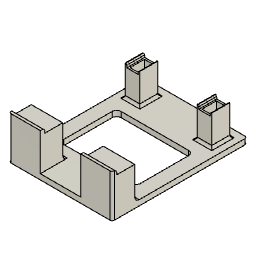
Header-Assembly-Jig (Autodesk Fusion 360 design; units mm, degrees)
Autodesk Fusion 360 part; units mm, degrees
sketch "Sketch1" plane through (0, 0, 0) normal (0, 0, 1) x (1, 0, 0)
  line L0 (1.9, -3.2) -> (-1.9, -3.2)
  line L1 (-1.9, -3.2) -> (-1.9, 3.2)
  line L2 (-1.9, 3.2) -> (1.9, 3.2)
  line L3 (1.9, 3.2) -> (1.9, -3.2)
  line L4 (1.9, -3.2) -> (-1.9, 3.2) construction
  line L5 (-1.9, -3.2) -> (1.9, 3.2) construction
  line L6 (2.55, -4) -> (-2.55, -4)
  line L7 (-2.55, -4) -> (-2.55, 4)
  line L8 (-2.55, 4) -> (2.55, 4)
  line L9 (2.55, 4) -> (2.55, -4)
  line L10 (2.55, -4) -> (-2.55, 4) construction
  line L11 (-2.55, -4) -> (2.55, 4) construction
  line L12 (3.25, -4) -> (-3.25, -4)
  line L13 (-3.25, -4) -> (-3.25, 4)
  line L14 (-3.25, 4) -> (3.25, 4)
  line L15 (3.25, 4) -> (3.25, -4)
  line L16 (3.25, -4) -> (-3.25, 4) construction
  line L17 (-3.25, -4) -> (3.25, 4) construction
  dimension "d1" = 3.8
  dimension "d2" = 6.4
  dimension "d3" = 5.1
  dimension "d4" = 8
  dimension "d5" = 6.5
  dimension "d6" = 8
  constraint horizontal L0
  constraint perpendicular L0 L1
  constraint parallel L0 L2
  constraint parallel L1 L3
  constraint coincident L4 origin
  constraint coincident L5 origin
  constraint horizontal L6
  constraint perpendicular L6 L7
  constraint parallel L6 L8
  constraint parallel L7 L9
  constraint coincident L10 origin
  constraint coincident L11 origin
  constraint horizontal L12
  constraint perpendicular L12 L13
  constraint parallel L12 L14
  constraint parallel L13 L15
  constraint coincident L16 origin
  constraint coincident L17 origin
  measures "d1" distance of L1.end L2.end
  measures "d2" distance of L0.end L1.end
  measures "d3" distance of L7.end L8.end
  measures "d4" distance of L6.end L7.end
  measures "d5" distance of L13.end L14.end
  measures "d6" distance of L12.end L13.end
extrude "Extrude1" add sketch "Sketch1" along normal blind 1.5 contours L9 L12 L14 L15 | L7 L12 L13 L14 makes body 1 at (3.25, 1.3333, 0.5) makes body 2 at (-3.25, -1.3333, 0.5)
extrude "Extrude2" add sketch "Sketch1" against normal blind 8 bodies 1 2
chamfer "Chamfer1" distance 0.5 angle 45 2 edges at (-2.55, 0, 1.5) (2.55, 0, 1.5) on bodies 1
sketch "Sketch2" plane through (0, 0, -8) normal (0, 0, -1) x (1, 0, 0)
  line L0 (1.9, -3.2) -> (-1.9, -3.2)
  line L1 (-1.9, -3.2) -> (-1.9, 3.2)
  line L2 (-1.9, 3.2) -> (1.9, 3.2)
  line L3 (1.9, 3.2) -> (1.9, -3.2)
  line L4 (-3.25, -4) -> (3.25, -4)
  line L5 (3.25, -4) -> (3.25, 4)
  line L6 (3.25, 4) -> (-3.25, 4)
  line L7 (-3.25, 4) -> (-3.25, -4)
  line L8 (3.25, -4) -> (-3.25, -4)
  line L9 (-3.25, -4) -> (-3.25, 4)
  line L10 (-3.25, 4) -> (3.25, 4)
  line L11 (3.25, 4) -> (3.25, -4)
  line L12 (3.25, -4) -> (-3.25, 4) construction
  line L13 (-3.25, -4) -> (3.25, 4) construction
  constraint horizontal L8
  constraint perpendicular L8 L9
  constraint parallel L8 L10
  constraint parallel L9 L11
  constraint coincident L4.end L5.start
  constraint coincident L12 origin
  constraint coincident L13 origin
extrude "Extrude3" add sketch "Sketch2" along normal blind 4 contours L0 L1 L2 L3 | L4 L5 L6 L7 L8 L9 L10 L11 bodies 1
sketch "Sketch3" plane through (0, 0, -12) normal (0, 0, -1) x (1, 0, 0)
  line L0 (3.25, 4) -> (-3.25, 4)
  line L1 (-3.25, 4) -> (-3.25, -4)
  line L2 (-3.25, -4) -> (3.25, -4)
  line L3 (3.25, -4) -> (3.25, 4)
  line L4 (-7, -8) -> (7, -8)
  line L5 (7, -8) -> (7, 50)
  line L6 (7, 50) -> (-7, 50)
  line L7 (-7, 50) -> (-7, -8)
  line L8 (-7, 50) -> (7, 50)
  line L9 (7, 50) -> (7, 42)
  line L10 (7, 42) -> (-7, 42)
  line L11 (-7, 42) -> (-7, 50)
  dimension "d14" = 14
  dimension "d15" = 58
  dimension "d16" = 4
  dimension "d20" = 8
  constraint horizontal L4
  constraint vertical L5
  constraint horizontal L6
  constraint vertical L7
  constraint horizontal L8
  constraint vertical L9
  constraint horizontal L10
  constraint vertical L11
  measures "d14" distance of L4.start L4.end
  measures "d15" distance of L4.start L6.end
  measures "d16" distance of L2 L4
  measures "d20" distance of L5.end L9.end
extrude "Extrude4" add sketch "Sketch3" along normal blind 2.4 separate body contours L0 L1 L2 L3 | L4 L5 L7 L10 | L5 L6 L7 L8 L9 L10 L11 makes body 3
extrude "Extrude5" add sketch "Sketch3" against normal blind 14.6 contours L5 L6 L7 L8 L9 L10 L11 bodies 3
move_face "OffsetFaces1" offset 2 1 faces at (2.3333, -50, -3.0667) on bodies 3
sketch "Sketch4" plane through (0, 0, 2.6) normal (0, 0, 1) x (-1, 0, 0)
  line L0 (-7, 42) -> (7, 42)
  line L1 (7, 42) -> (7, 52)
  line L2 (7, 52) -> (-7, 52)
  line L3 (-7, 52) -> (-7, 42)
  line L4 (7, 52) -> (-7, 52)
  line L5 (-7, 52) -> (-7, 50)
  line L6 (-7, 50) -> (7, 50)
  line L7 (7, 50) -> (7, 52)
  dimension "d24" = 14
  dimension "d25" = 2
  constraint horizontal L4
  constraint vertical L5
  constraint horizontal L6
  constraint vertical L7
  constraint coincident L1.end L2.start
  measures "d24" distance of L1.end L2.end
  measures "d25" distance of L1.end L6.end
extrude "Extrude6" add sketch "Sketch4" along normal blind 2 contours L1 L2 L3 L4 L5 L6 L7 bodies 3
chamfer "Chamfer2" distance 0.8 angle 45 1 edges at (0, -50, 4.6) on bodies 3
fillet "Fillet1" radius 2 1 edges at (0, -42, -12) on bodies 3
fillet "Fillet2" [suppressed]
combine "Combine1" operation add target body 3 tool bodies 1
fillet "Fillet3" radius 1 4 edges at (0, 4, -12) (3.25, 0, -12) (0, -4, -12) (-3.25, 0, -12) on bodies 3
copy_body "CopyPasteBodies1" bodies 3 makes body 4
move_body "Move1" bodies 4 to x (1, 0, 0) y (0, 1, 0) z (0, 0, 1) at (-32, 0, 0)
sketch "Sketch5" plane through (0, 0, -14.4) normal (0, 0, -1) x (1, 0, 0)
  line L0 (-7, -8) -> (7, -8)
  line L1 (7, -8) -> (7, 52)
  line L2 (7, 52) -> (-7, 52)
  line L3 (-7, 52) -> (-7, -8)
  line L4 (-39, 52) -> (7, 52)
  line L5 (7, 52) -> (7, -8)
  line L6 (7, -8) -> (-39, -8)
  line L7 (-39, -8) -> (-39, 52)
  constraint horizontal L4
  constraint vertical L5
  constraint horizontal L6
  constraint vertical L7
  constraint coincident L0.end L1.start
extrude "Extrude7" add sketch "Sketch5" against normal blind 2.4 contours L3 L4 L6 L7 bodies 4 3
sketch "Sketch6" plane through (0, 0, -12) normal (0, 0, 1) x (-1, 0, 0)
  line L0 (4.25, -5) -> (-4.25, -5)
  line L1 (-4.25, -5) -> (-4.25, 5)
  line L2 (-4.25, 5) -> (4.25, 5)
  line L3 (4.25, 5) -> (4.25, -5)
  line L4 (39, 40) -> (25, 40)
  line L5 (25, 40) -> (25, 52)
  line L6 (25, 52) -> (7, 52)
  line L7 (7, 52) -> (7, 40)
  line L8 (7, 40) -> (-7, 40)
  line L9 (-7, 40) -> (-7, -8)
  line L10 (-7, -8) -> (39, -8)
  line L11 (39, -8) -> (39, 40)
  line L12 (36.25, -5) -> (27.75, -5)
  line L13 (27.75, -5) -> (27.75, 5)
  line L14 (27.75, 5) -> (36.25, 5)
  line L15 (36.25, 5) -> (36.25, -5)
  line L16 (-1, 35.5269) -> (33, 35.5269)
  line L17 (33, 35.5269) -> (33, 10.0468)
  line L18 (33, 10.0468) -> (-1, 10.0468)
  line L19 (-1, 10.0468) -> (-1, 35.5269)
  line L20 (-1, 35.5269) -> (33, 10.0468) construction
  line L21 (33, 35.5269) -> (-1, 10.0468) construction
  point P0 (16, 22.7869)
  constraint horizontal L16
  constraint perpendicular L16 L17
  constraint parallel L16 L18
  constraint parallel L17 L19
  constraint coincident L20 P0
  constraint coincident L21 P0
  constraint midpoint L21 P0
extrude "Extrude8" cut sketch "Sketch6" against normal up to surface (2.4 mm away) contours L16 L17 L18 L19 bodies 4
fillet "Fillet4" radius 2 4 edges at (1, -35.5269, -13.2) (-33, -35.5269, -13.2) (-33, -10.0468, -13.2) (1, -10.0468, -13.2) on bodies 4
fillet "Fillet5" radius 1 4 edges at (-39, -52, -4.9) (7, -52, -4.9) (-39, 8, -13.2) (7, 8, -13.2) on bodies 4
